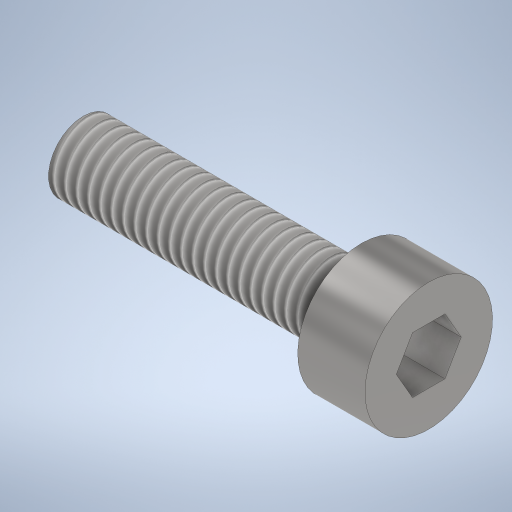
# Autodesk Inventor part: fasten_bolt
Saved by Autodesk Inventor 2023 (Build 270158000, 158)
## iProperties
Created: 2023-03-26
Part Number: fasten_bolt
Material: Steel, Mild
Document SubType Name: Modeling
Designer: maste
Density: 7.85 g/cm^3
Appearance: Semi-Polished
Author: maste
Autodesk Inventor part; units mm, degrees
ref_plane "YZ Plane" through (0, 0, 0) normal (1, 0, 0) x (0, 1, 0)
ref_plane "XZ Plane" through (0, 0, 0) normal (0, 1, 0) x (-1, 0, 0)
ref_plane "XY Plane" through (0, 0, 0) normal (0, 0, 1) x (1, 0, 0)
sketch "Sketch1" plane through (0, 0, 0) normal (0, 0, 1) x (1, 0, 0)
  line L0 (0, 0) -> (14.9, 0)
  line L1 (14.9, 0) -> (14.9, 2.75)
  line L2 (14.9, 2.75) -> (12, 2.75)
  line L3 (0, 0) -> (0, 1.5)
  line L4 (0, 1.5) -> (12, 1.5)
  line L5 (12, 1.5) -> (12, 2.75)
  dimension "d0" = 14.9
  dimension "d1" = 2.75
  dimension "d2" = 2.9
  dimension "d3" = 1.5
  constraints: 12 end point, 4 perpendicular, 1 horizontal, 1 vertical
  measures "d0" distance of L0.start L0.end
  measures "d1" distance of L0.end L1.end
  measures "d2" distance of L1.end L2.end
  measures "d3" distance of L0.start L3.end
revolve "Revolution1" add sketch "Sketch1" angle 360 about axis through (0, 0, 0) along (1, 0, 0)
sketch "Sketch2" plane through (14.9, 0, 0) normal (1, 0, 0) x (0, 0, -1)
  line L0 (0.7, 1.2124) -> (1.4, 0)
  line L1 (1.4, 0) -> (0.7, -1.2124)
  line L2 (0.7, -1.2124) -> (-0.7, -1.2124)
  line L3 (-0.7, -1.2124) -> (-1.4, 0)
  line L4 (-1.4, 0) -> (-0.7, 1.2124)
  line L5 (-0.7, 1.2124) -> (0.7, 1.2124)
  point P0 (0, 0)
  point P1 (0, 0)
  dimension "d6" = 2.8
  constraints: 12 end point, 1 coincident, 13 other
  measures "d6" distance of L0.end L3.end
extrude "Extrusion1" cut sketch "Sketch2" against normal blind 1.9
thread "Thread1" size "M3x0.5" class "6g" standard "ANSI Metric M Profile" full length
body "Solid1"
